Autodesk Fusion 360 part; units mm, degrees
note: some values were not read from the file. Chosen so that the rebuilt part matches the saved one: a direction. Set by a fixed rule: which sketch regions a step uses; which face or edge a step refers to.
(part 3 of 6)
  spline S532 degree 3 poles (194.827, -53.1151) (193.9004, -54.7201) (192.568, -56.0525) (190.963, -56.9791) knots 0 0 0 0 1 1 1 1
  spline S533 degree 3 poles (190.963, -56.9791) (189.3581, -57.9057) (187.5377, -58.3935) (185.6846, -58.3935) knots 0 0 0 0 1 1 1 1
  line L538 (185.6846, -58.3935) -> (156.5804, -58.3935)
  spline S534 degree 3 poles (156.5804, -58.3935) (156.5659, -58.3935) (156.554, -58.4054) (156.554, -58.42) knots 0 0 0 0 1 1 1 1
  line L539 (156.554, -58.42) -> (156.554, -59.2138)
  spline S535 degree 3 poles (156.554, -59.2138) (156.554, -59.2283) (156.5659, -59.2402) (156.5804, -59.2402) knots 0 0 0 0 1 1 1 1
  line L540 (155.3369, -57.9967) -> (184.441, -57.9967)
  spline S536 degree 3 poles (184.441, -57.9967) (186.4429, -57.9967) (188.4093, -57.4699) (190.1428, -56.469) knots 0 0 0 0 1 1 1 1
  spline S537 degree 3 poles (190.1428, -56.469) (191.8764, -55.468) (193.316, -54.0284) (194.3169, -52.2949) knots 0 0 0 0 1 1 1 1
  spline S538 degree 3 poles (194.3169, -52.2949) (195.3178, -50.5613) (195.8446, -48.595) (195.8446, -46.5931) knots 0 0 0 0 1 1 1 1
  spline S539 degree 3 poles (195.8446, -46.5931) (195.8446, -46.5786) (195.8327, -46.5667) (195.8181, -46.5667) knots 0 0 0 0 1 1 1 1
  line L541 (195.8181, -46.5667) -> (195.0244, -46.5667)
  spline S540 degree 3 poles (195.0244, -46.5667) (195.0098, -46.5667) (194.9979, -46.5786) (194.9979, -46.5931) knots 0 0 0 0 1 1 1 1
  spline S541 degree 3 poles (194.9979, -46.5931) (194.9979, -48.4463) (194.51, -50.2666) (193.5835, -51.8716) knots 0 0 0 0 1 1 1 1
  spline S542 degree 3 poles (193.5835, -51.8716) (192.6569, -53.4765) (191.3244, -54.809) (189.7195, -55.7355) knots 0 0 0 0 1 1 1 1
  spline S543 degree 3 poles (189.7195, -55.7355) (188.1145, -56.6621) (186.2942, -57.15) (184.441, -57.15) knots 0 0 0 0 1 1 1 1
  line L542 (184.441, -57.15) -> (155.3369, -57.15)
  spline S544 degree 3 poles (155.3369, -57.15) (155.3223, -57.15) (155.3104, -57.1619) (155.3104, -57.1765) knots 0 0 0 0 1 1 1 1
  line L543 (155.3104, -57.1765) -> (155.3104, -57.9702)
  spline S545 degree 3 poles (155.3104, -57.9702) (155.3104, -57.9848) (155.3223, -57.9967) (155.3369, -57.9967) knots 0 0 0 0 1 1 1 1
  line L544 (155.7337, -56.7531) -> (184.8379, -56.7531)
  spline S546 degree 3 poles (184.8379, -56.7531) (186.4913, -56.7531) (188.1156, -56.3179) (189.5475, -55.4913) knots 0 0 0 0 1 1 1 1
  spline S547 degree 3 poles (189.5475, -55.4913) (190.9794, -54.6645) (192.1685, -53.4755) (192.9953, -52.0435) knots 0 0 0 0 1 1 1 1
  spline S548 degree 3 poles (192.9953, -52.0435) (193.8218, -50.6116) (194.2571, -48.9873) (194.2571, -47.334) knots 0 0 0 0 1 1 1 1
  spline S549 degree 3 poles (194.2571, -47.334) (194.2571, -47.3194) (194.2452, -47.3075) (194.2306, -47.3075) knots 0 0 0 0 1 1 1 1
  line L545 (194.2306, -47.3075) -> (193.4369, -47.3075)
  spline S550 degree 3 poles (193.4369, -47.3075) (193.4223, -47.3075) (193.4104, -47.3194) (193.4104, -47.334) knots 0 0 0 0 1 1 1 1
  spline S551 degree 3 poles (193.4104, -47.334) (193.4104, -48.8386) (193.0143, -50.3171) (192.2619, -51.6202) knots 0 0 0 0 1 1 1 1
  spline S552 degree 3 poles (192.2619, -51.6202) (191.5096, -52.9233) (190.4272, -54.0057) (189.1242, -54.7579) knots 0 0 0 0 1 1 1 1
  spline S553 degree 3 poles (189.1242, -54.7579) (187.8211, -55.5104) (186.3426, -55.9065) (184.8379, -55.9065) knots 0 0 0 0 1 1 1 1
  line L546 (184.8379, -55.9065) -> (155.7337, -55.9065)
  spline S554 degree 3 poles (155.7337, -55.9065) (155.7192, -55.9065) (155.7073, -55.9184) (155.7073, -55.9329) knots 0 0 0 0 1 1 1 1
  line L547 (155.7073, -55.9329) -> (155.7073, -56.7267)
  spline S555 degree 3 poles (155.7073, -56.7267) (155.7073, -56.7412) (155.7192, -56.7531) (155.7337, -56.7531) knots 0 0 0 0 1 1 1 1
  line L548 (154.4902, -55.5096) -> (183.5944, -55.5096)
  spline S556 degree 3 poles (183.5944, -55.5096) (185.2478, -55.5096) (186.872, -55.0743) (188.304, -54.2478) knots 0 0 0 0 1 1 1 1
  spline S557 degree 3 poles (188.304, -54.2478) (189.7359, -53.421) (190.9249, -52.2319) (191.7517, -50.8) knots 0 0 0 0 1 1 1 1
  spline S558 degree 3 poles (191.7517, -50.8) (192.5783, -49.3681) (193.0135, -47.7438) (193.0135, -46.0904) knots 0 0 0 0 1 1 1 1
  spline S559 degree 3 poles (193.0135, -46.0904) (193.0135, -46.0759) (193.0016, -46.064) (192.9871, -46.064) knots 0 0 0 0 1 1 1 1
  line L549 (192.9871, -46.064) -> (192.1933, -46.064)
  spline S560 degree 3 poles (192.1933, -46.064) (192.1788, -46.064) (192.1669, -46.0759) (192.1669, -46.0904) knots 0 0 0 0 1 1 1 1
  spline S561 degree 3 poles (192.1669, -46.0904) (192.1669, -47.5951) (191.7708, -49.0736) (191.0183, -50.3767) knots 0 0 0 0 1 1 1 1
  spline S562 degree 3 poles (191.0183, -50.3767) (190.2661, -51.6797) (189.1837, -52.7622) (187.8806, -53.5144) knots 0 0 0 0 1 1 1 1
  spline S563 degree 3 poles (187.8806, -53.5144) (186.5775, -54.2668) (185.0991, -54.6629) (183.5944, -54.6629) knots 0 0 0 0 1 1 1 1
  line L550 (183.5944, -54.6629) -> (154.4902, -54.6629)
  spline S564 degree 3 poles (154.4902, -54.6629) (154.4756, -54.6629) (154.4637, -54.6748) (154.4637, -54.6894) knots 0 0 0 0 1 1 1 1
  line L551 (154.4637, -54.6894) -> (154.4637, -55.4831)
  spline S565 degree 3 poles (154.4637, -55.4831) (154.4637, -55.4977) (154.4756, -55.5096) (154.4902, -55.5096) knots 0 0 0 0 1 1 1 1
  line L552 (3.466, -30.7446) -> (5.0535, -30.7446)
  spline S566 degree 3 poles (5.0535, -30.7446) (5.0681, -30.7446) (5.08, -30.7327) (5.08, -30.7181) knots 0 0 0 0 1 1 1 1
  line L553 (5.08, -30.7181) -> (5.08, -29.9508)
  spline S567 degree 3 poles (5.08, -29.9508) (5.08, -29.9244) (5.0535, -29.9508) (5.08, -29.9508) knots 0 0 0 0 1 1 1 1
  line L554 (5.08, -29.9508) -> (6.6146, -29.9508)
  spline S568 degree 3 poles (6.6146, -29.9508) (6.641, -29.9508) (6.6146, -29.9244) (6.6146, -29.9508) knots 0 0 0 0 1 1 1 1
  line L555 (6.6146, -29.9508) -> (6.6146, -30.7181)
  spline S569 degree 3 poles (6.6146, -30.7181) (6.6146, -30.7327) (6.6265, -30.7446) (6.641, -30.7446) knots 0 0 0 0 1 1 1 1
  line L556 (6.641, -30.7446) -> (8.2285, -30.7446)
  spline S570 degree 3 poles (8.2285, -30.7446) (8.2431, -30.7446) (8.255, -30.7327) (8.255, -30.7181) knots 0 0 0 0 1 1 1 1
  line L557 (8.255, -30.7181) -> (8.255, -29.9508)
  spline S571 degree 3 poles (8.255, -29.9508) (8.255, -29.9244) (8.2285, -29.9508) (8.255, -29.9508) knots 0 0 0 0 1 1 1 1
  line L558 (8.255, -29.9508) -> (9.7896, -29.9508)
  spline S572 degree 3 poles (9.7896, -29.9508) (9.816, -29.9508) (9.7896, -29.9244) (9.7896, -29.9508) knots 0 0 0 0 1 1 1 1
  line L559 (9.7896, -29.9508) -> (9.7896, -30.7181)
  spline S573 degree 3 poles (9.7896, -30.7181) (9.7896, -30.7327) (9.8015, -30.7446) (9.816, -30.7446) knots 0 0 0 0 1 1 1 1
  line L560 (9.816, -30.7446) -> (11.4035, -30.7446)
  spline S574 degree 3 poles (11.4035, -30.7446) (11.4181, -30.7446) (11.43, -30.7327) (11.43, -30.7181) knots 0 0 0 0 1 1 1 1
  line L561 (11.43, -30.7181) -> (11.43, -29.9508)
  spline S575 degree 3 poles (11.43, -29.9508) (11.43, -29.9244) (11.4035, -29.9508) (11.43, -29.9508) knots 0 0 0 0 1 1 1 1
  line L562 (11.43, -29.9508) -> (12.9646, -29.9508)
  spline S576 degree 3 poles (12.9646, -29.9508) (12.991, -29.9508) (12.9646, -29.9244) (12.9646, -29.9508) knots 0 0 0 0 1 1 1 1
  line L563 (12.9646, -29.9508) -> (12.9646, -30.7181)
  spline S577 degree 3 poles (12.9646, -30.7181) (12.9646, -30.7327) (12.9765, -30.7446) (12.991, -30.7446) knots 0 0 0 0 1 1 1 1
  line L564 (12.991, -30.7446) -> (14.5785, -30.7446)
  spline S578 degree 3 poles (14.5785, -30.7446) (14.5931, -30.7446) (14.605, -30.7327) (14.605, -30.7181) knots 0 0 0 0 1 1 1 1
  line L565 (14.605, -30.7181) -> (14.605, -29.9508)
  spline S579 degree 3 poles (14.605, -29.9508) (14.605, -29.9244) (14.5785, -29.9508) (14.605, -29.9508) knots 0 0 0 0 1 1 1 1
  line L566 (14.605, -29.9508) -> (16.1396, -29.9508)
  spline S580 degree 3 poles (16.1396, -29.9508) (16.166, -29.9508) (16.1396, -29.9244) (16.1396, -29.9508) knots 0 0 0 0 1 1 1 1
  line L567 (16.1396, -29.9508) -> (16.1396, -30.7181)
  spline S581 degree 3 poles (16.1396, -30.7181) (16.1396, -30.7327) (16.1515, -30.7446) (16.166, -30.7446) knots 0 0 0 0 1 1 1 1
  line L568 (16.166, -30.7446) -> (17.7535, -30.7446)
  spline S582 degree 3 poles (17.7535, -30.7446) (17.7681, -30.7446) (17.78, -30.7327) (17.78, -30.7181) knots 0 0 0 0 1 1 1 1
  line L569 (17.78, -30.7181) -> (17.78, -29.9508)
  spline S583 degree 3 poles (17.78, -29.9508) (17.78, -29.9244) (17.7535, -29.9508) (17.78, -29.9508) knots 0 0 0 0 1 1 1 1
  line L570 (17.78, -29.9508) -> (19.3146, -29.9508)
  spline S584 degree 3 poles (19.3146, -29.9508) (19.341, -29.9508) (19.3146, -29.9244) (19.3146, -29.9508) knots 0 0 0 0 1 1 1 1
  line L571 (19.3146, -29.9508) -> (19.3146, -30.7181)
  spline S585 degree 3 poles (19.3146, -30.7181) (19.3146, -30.7327) (19.3265, -30.7446) (19.341, -30.7446) knots 0 0 0 0 1 1 1 1
  line L572 (19.341, -30.7446) -> (20.9285, -30.7446)
  spline S586 degree 3 poles (20.9285, -30.7446) (20.9431, -30.7446) (20.955, -30.7327) (20.955, -30.7181) knots 0 0 0 0 1 1 1 1
  line L573 (20.955, -30.7181) -> (20.955, -29.9508)
  spline S587 degree 3 poles (20.955, -29.9508) (20.955, -29.9244) (20.9285, -29.9508) (20.955, -29.9508) knots 0 0 0 0 1 1 1 1
  line L574 (20.955, -29.9508) -> (22.4896, -29.9508)
  spline S588 degree 3 poles (22.4896, -29.9508) (22.516, -29.9508) (22.4896, -29.9244) (22.4896, -29.9508) knots 0 0 0 0 1 1 1 1
  line L575 (22.4896, -29.9508) -> (22.4896, -30.7181)
  spline S589 degree 3 poles (22.4896, -30.7181) (22.4896, -30.7327) (22.5015, -30.7446) (22.516, -30.7446) knots 0 0 0 0 1 1 1 1
  line L576 (22.516, -30.7446) -> (24.1035, -30.7446)
  spline S590 degree 3 poles (24.1035, -30.7446) (24.1181, -30.7446) (24.13, -30.7327) (24.13, -30.7181) knots 0 0 0 0 1 1 1 1
  line L577 (24.13, -30.7181) -> (24.13, -29.9508)
  spline S591 degree 3 poles (24.13, -29.9508) (24.13, -29.9244) (24.1035, -29.9508) (24.13, -29.9508) knots 0 0 0 0 1 1 1 1
  line L578 (24.13, -29.9508) -> (25.6646, -29.9508)
  spline S592 degree 3 poles (25.6646, -29.9508) (25.691, -29.9508) (25.6646, -29.9244) (25.6646, -29.9508) knots 0 0 0 0 1 1 1 1
  line L579 (25.6646, -29.9508) -> (25.6646, -30.7181)
  spline S593 degree 3 poles (25.6646, -30.7181) (25.6646, -30.7327) (25.6765, -30.7446) (25.691, -30.7446) knots 0 0 0 0 1 1 1 1
  line L580 (25.691, -30.7446) -> (27.2785, -30.7446)
  spline S594 degree 3 poles (27.2785, -30.7446) (27.2931, -30.7446) (27.305, -30.7327) (27.305, -30.7181) knots 0 0 0 0 1 1 1 1
  line L581 (27.305, -30.7181) -> (27.305, -29.9508)
  spline S595 degree 3 poles (27.305, -29.9508) (27.305, -29.9244) (27.2785, -29.9508) (27.305, -29.9508) knots 0 0 0 0 1 1 1 1
  line L582 (27.305, -29.9508) -> (28.8396, -29.9508)
  spline S596 degree 3 poles (28.8396, -29.9508) (28.866, -29.9508) (28.8396, -29.9244) (28.8396, -29.9508) knots 0 0 0 0 1 1 1 1
  line L583 (28.8396, -29.9508) -> (28.8396, -30.7181)
  spline S597 degree 3 poles (28.8396, -30.7181) (28.8396, -30.7327) (28.8515, -30.7446) (28.866, -30.7446) knots 0 0 0 0 1 1 1 1
  line L584 (28.866, -30.7446) -> (30.4535, -30.7446)
  spline S598 degree 3 poles (30.4535, -30.7446) (30.4681, -30.7446) (30.48, -30.7327) (30.48, -30.7181) knots 0 0 0 0 1 1 1 1
  line L585 (30.48, -30.7181) -> (30.48, -29.9508)
  spline S599 degree 3 poles (30.48, -29.9508) (30.48, -29.9244) (30.4535, -29.9508) (30.48, -29.9508) knots 0 0 0 0 1 1 1 1
  line L586 (30.48, -29.9508) -> (32.0146, -29.9508)
  spline S600 degree 3 poles (32.0146, -29.9508) (32.041, -29.9508) (32.0146, -29.9244) (32.0146, -29.9508) knots 0 0 0 0 1 1 1 1
  line L587 (32.0146, -29.9508) -> (32.0146, -30.7181)
  spline S601 degree 3 poles (32.0146, -30.7181) (32.0146, -30.7327) (32.0265, -30.7446) (32.041, -30.7446) knots 0 0 0 0 1 1 1 1
  line L588 (32.041, -30.7446) -> (33.6285, -30.7446)
  spline S602 degree 3 poles (33.6285, -30.7446) (33.6431, -30.7446) (33.655, -30.7327) (33.655, -30.7181) knots 0 0 0 0 1 1 1 1
  line L589 (33.655, -30.7181) -> (33.655, -29.9508)
  spline S603 degree 3 poles (33.655, -29.9508) (33.655, -29.9244) (33.6285, -29.9508) (33.655, -29.9508) knots 0 0 0 0 1 1 1 1
  line L590 (33.655, -29.9508) -> (35.1896, -29.9508)
  spline S604 degree 3 poles (35.1896, -29.9508) (35.216, -29.9508) (35.1896, -29.9244) (35.1896, -29.9508) knots 0 0 0 0 1 1 1 1
  line L591 (35.1896, -29.9508) -> (35.1896, -30.7181)
  spline S605 degree 3 poles (35.1896, -30.7181) (35.1896, -30.7327) (35.2015, -30.7446) (35.216, -30.7446) knots 0 0 0 0 1 1 1 1
  line L592 (35.216, -30.7446) -> (36.8035, -30.7446)
  spline S606 degree 3 poles (36.8035, -30.7446) (36.8181, -30.7446) (36.83, -30.7327) (36.83, -30.7181) knots 0 0 0 0 1 1 1 1
  line L593 (36.83, -30.7181) -> (36.83, -29.9508)
  spline S607 degree 3 poles (36.83, -29.9508) (36.83, -29.9244) (36.8035, -29.9508) (36.83, -29.9508) knots 0 0 0 0 1 1 1 1
  line L594 (36.83, -29.9508) -> (38.3646, -29.9508)
  spline S608 degree 3 poles (38.3646, -29.9508) (38.391, -29.9508) (38.3646, -29.9244) (38.3646, -29.9508) knots 0 0 0 0 1 1 1 1
  line L595 (38.3646, -29.9508) -> (38.3646, -30.7181)
  spline S609 degree 3 poles (38.3646, -30.7181) (38.3646, -30.7327) (38.3765, -30.7446) (38.391, -30.7446) knots 0 0 0 0 1 1 1 1
  line L596 (38.391, -30.7446) -> (39.9785, -30.7446)
  spline S610 degree 3 poles (39.9785, -30.7446) (39.9931, -30.7446) (40.005, -30.7327) (40.005, -30.7181) knots 0 0 0 0 1 1 1 1
  line L597 (40.005, -30.7181) -> (40.005, -29.9508)
  spline S611 degree 3 poles (40.005, -29.9508) (40.005, -29.9244) (39.9785, -29.9508) (40.005, -29.9508) knots 0 0 0 0 1 1 1 1
  line L598 (40.005, -29.9508) -> (41.5396, -29.9508)
  spline S612 degree 3 poles (41.5396, -29.9508) (41.566, -29.9508) (41.5396, -29.9244) (41.5396, -29.9508) knots 0 0 0 0 1 1 1 1
  line L599 (41.5396, -29.9508) -> (41.5396, -30.7181)
  spline S613 degree 3 poles (41.5396, -30.7181) (41.5396, -30.7327) (41.5515, -30.7446) (41.566, -30.7446) knots 0 0 0 0 1 1 1 1
  line L600 (41.566, -30.7446) -> (43.1535, -30.7446)
  line L601 (43.1535, -30.7446) -> (43.9473, -30.7446)
  spline S614 degree 3 poles (43.9473, -30.7446) (43.9618, -30.7446) (43.9737, -30.7327) (43.9737, -30.7181) knots 0 0 0 0 1 1 1 1
  line L602 (43.9737, -30.7181) -> (43.9737, -29.9244)
  line L603 (43.9737, -29.9244) -> (43.9737, -28.6015)
  spline S615 degree 3 poles (43.9737, -28.6015) (43.9737, -28.5869) (43.9618, -28.575) (43.9473, -28.575) knots 0 0 0 0 1 1 1 1
  line L604 (43.9473, -28.575) -> (43.18, -28.575)
  spline S616 degree 3 poles (43.18, -28.575) (43.1535, -28.575) (43.18, -28.6015) (43.18, -28.575) knots 0 0 0 0 1 1 1 1
  line L605 (43.18, -28.575) -> (43.18, -27.0404)
  spline S617 degree 3 poles (43.18, -27.0404) (43.18, -27.014) (43.1535, -27.0404) (43.18, -27.0404) knots 0 0 0 0 1 1 1 1
  line L606 (43.18, -27.0404) -> (43.9473, -27.0404)
  spline S618 degree 3 poles (43.9473, -27.0404) (43.9618, -27.0404) (43.9737, -27.0285) (43.9737, -27.014) knots 0 0 0 0 1 1 1 1
  line L607 (43.9737, -27.014) -> (43.9737, -25.4265)
  spline S619 degree 3 poles (43.9737, -25.4265) (43.9737, -25.4119) (43.9618, -25.4) (43.9473, -25.4) knots 0 0 0 0 1 1 1 1
  line L608 (43.9473, -25.4) -> (43.18, -25.4)
  spline S620 degree 3 poles (43.18, -25.4) (43.1535, -25.4) (43.18, -25.4265) (43.18, -25.4) knots 0 0 0 0 1 1 1 1
  line L609 (43.18, -25.4) -> (43.18, -23.8654)
  spline S621 degree 3 poles (43.18, -23.8654) (43.18, -23.839) (43.1535, -23.8654) (43.18, -23.8654) knots 0 0 0 0 1 1 1 1
  line L610 (43.18, -23.8654) -> (43.9473, -23.8654)
  spline S622 degree 3 poles (43.9473, -23.8654) (43.9618, -23.8654) (43.9737, -23.8535) (43.9737, -23.839) knots 0 0 0 0 1 1 1 1
  line L611 (43.9737, -23.839) -> (43.9737, -22.2515)
  spline S623 degree 3 poles (43.9737, -22.2515) (43.9737, -22.2369) (43.9618, -22.225) (43.9473, -22.225) knots 0 0 0 0 1 1 1 1
  line L612 (43.9473, -22.225) -> (43.18, -22.225)
  spline S624 degree 3 poles (43.18, -22.225) (43.1535, -22.225) (43.18, -22.2515) (43.18, -22.225) knots 0 0 0 0 1 1 1 1
  line L613 (43.18, -22.225) -> (43.18, -20.6904)
  spline S625 degree 3 poles (43.18, -20.6904) (43.18, -20.664) (43.1535, -20.6904) (43.18, -20.6904) knots 0 0 0 0 1 1 1 1
  line L614 (43.18, -20.6904) -> (43.9473, -20.6904)
  spline S626 degree 3 poles (43.9473, -20.6904) (43.9618, -20.6904) (43.9737, -20.6785) (43.9737, -20.664) knots 0 0 0 0 1 1 1 1
  line L615 (43.9737, -20.664) -> (43.9737, -19.0765)
  spline S627 degree 3 poles (43.9737, -19.0765) (43.9737, -19.0619) (43.9618, -19.05) (43.9473, -19.05) knots 0 0 0 0 1 1 1 1
  line L616 (43.9473, -19.05) -> (43.18, -19.05)
  spline S628 degree 3 poles (43.18, -19.05) (43.1535, -19.05) (43.18, -19.0765) (43.18, -19.05) knots 0 0 0 0 1 1 1 1
  line L617 (43.18, -19.05) -> (43.18, -17.5154)
  spline S629 degree 3 poles (43.18, -17.5154) (43.18, -17.489) (43.1535, -17.5154) (43.18, -17.5154) knots 0 0 0 0 1 1 1 1
  line L618 (43.18, -17.5154) -> (43.9473, -17.5154)
  spline S630 degree 3 poles (43.9473, -17.5154) (43.9618, -17.5154) (43.9737, -17.5035) (43.9737, -17.489) knots 0 0 0 0 1 1 1 1
  line L619 (43.9737, -17.489) -> (43.9737, -15.9015)
  spline S631 degree 3 poles (43.9737, -15.9015) (43.9737, -15.8869) (43.9618, -15.875) (43.9473, -15.875) knots 0 0 0 0 1 1 1 1
  line L620 (43.9473, -15.875) -> (43.18, -15.875)
  spline S632 degree 3 poles (43.18, -15.875) (43.1535, -15.875) (43.18, -15.9015) (43.18, -15.875) knots 0 0 0 0 1 1 1 1
  line L621 (43.18, -15.875) -> (43.18, -14.3404)
  spline S633 degree 3 poles (43.18, -14.3404) (43.18, -14.314) (43.1535, -14.3404) (43.18, -14.3404) knots 0 0 0 0 1 1 1 1
  line L622 (43.18, -14.3404) -> (43.9473, -14.3404)
  spline S634 degree 3 poles (43.9473, -14.3404) (43.9618, -14.3404) (43.9737, -14.3285) (43.9737, -14.314) knots 0 0 0 0 1 1 1 1
  line L623 (43.9737, -14.314) -> (43.9737, -12.7265)
  spline S635 degree 3 poles (43.9737, -12.7265) (43.9737, -12.7119) (43.9618, -12.7) (43.9473, -12.7) knots 0 0 0 0 1 1 1 1
  line L624 (43.9473, -12.7) -> (43.18, -12.7)
  spline S636 degree 3 poles (43.18, -12.7) (43.1535, -12.7) (43.18, -12.7265) (43.18, -12.7) knots 0 0 0 0 1 1 1 1
  line L625 (43.18, -12.7) -> (43.18, -11.1654)
  spline S637 degree 3 poles (43.18, -11.1654) (43.18, -11.139) (43.1535, -11.1654) (43.18, -11.1654) knots 0 0 0 0 1 1 1 1
  line L626 (43.18, -11.1654) -> (43.9473, -11.1654)
  spline S638 degree 3 poles (43.9473, -11.1654) (43.9618, -11.1654) (43.9737, -11.1535) (43.9737, -11.139) knots 0 0 0 0 1 1 1 1
  line L627 (43.9737, -11.139) -> (43.9737, -9.5515)
  spline S639 degree 3 poles (43.9737, -9.5515) (43.9737, -9.5369) (43.9618, -9.525) (43.9473, -9.525) knots 0 0 0 0 1 1 1 1
  line L628 (43.9473, -9.525) -> (43.18, -9.525)
  spline S640 degree 3 poles (43.18, -9.525) (43.1535, -9.525) (43.18, -9.5515) (43.18, -9.525) knots 0 0 0 0 1 1 1 1
  line L629 (43.18, -9.525) -> (43.18, -7.9904)
  spline S641 degree 3 poles (43.18, -7.9904) (43.18, -7.964) (43.1535, -7.9904) (43.18, -7.9904) knots 0 0 0 0 1 1 1 1
  line L630 (43.18, -7.9904) -> (43.9473, -7.9904)
  spline S642 degree 3 poles (43.9473, -7.9904) (43.9618, -7.9904) (43.9737, -7.9785) (43.9737, -7.964) knots 0 0 0 0 1 1 1 1
  line L631 (43.9737, -7.964) -> (43.9737, -6.3765)
  spline S643 degree 3 poles (43.9737, -6.3765) (43.9737, -6.3619) (43.9618, -6.35) (43.9473, -6.35) knots 0 0 0 0 1 1 1 1
  line L632 (43.9473, -6.35) -> (43.18, -6.35)
  spline S644 degree 3 poles (43.18, -6.35) (43.1535, -6.35) (43.18, -6.3765) (43.18, -6.35) knots 0 0 0 0 1 1 1 1
  line L633 (43.18, -6.35) -> (43.18, -4.8154)
  spline S645 degree 3 poles (43.18, -4.8154) (43.18, -4.789) (43.1535, -4.8154) (43.18, -4.8154) knots 0 0 0 0 1 1 1 1
  line L634 (43.18, -4.8154) -> (43.9473, -4.8154)
  spline S646 degree 3 poles (43.9473, -4.8154) (43.9618, -4.8154) (43.9737, -4.8035) (43.9737, -4.789) knots 0 0 0 0 1 1 1 1
  line L635 (43.9737, -4.789) -> (43.9737, -3.466)
  line L636 (43.9737, -3.466) -> (43.9737, -2.6723)
  spline S647 degree 3 poles (43.9737, -2.6723) (43.9737, -2.6577) (43.9618, -2.6458) (43.9473, -2.6458) knots 0 0 0 0 1 1 1 1
  line L637 (43.9473, -2.6458) -> (43.1535, -2.6458)
  line L638 (43.1535, -2.6458) -> (41.566, -2.6458)
  spline S648 degree 3 poles (41.566, -2.6458) (41.5515, -2.6458) (41.5396, -2.6577) (41.5396, -2.6723) knots 0 0 0 0 1 1 1 1
  line L639 (41.5396, -2.6723) -> (41.5396, -3.4396)
  spline S649 degree 3 poles (41.5396, -3.4396) (41.5396, -3.466) (41.566, -3.4396) (41.5396, -3.4396) knots 0 0 0 0 1 1 1 1
  line L640 (41.5396, -3.4396) -> (40.005, -3.4396)
  spline S650 degree 3 poles (40.005, -3.4396) (39.9785, -3.4396) (40.005, -3.466) (40.005, -3.4396) knots 0 0 0 0 1 1 1 1
  line L641 (40.005, -3.4396) -> (40.005, -2.6723)
  spline S651 degree 3 poles (40.005, -2.6723) (40.005, -2.6577) (39.9931, -2.6458) (39.9785, -2.6458) knots 0 0 0 0 1 1 1 1
  line L642 (39.9785, -2.6458) -> (38.391, -2.6458)
  spline S652 degree 3 poles (38.391, -2.6458) (38.3765, -2.6458) (38.3646, -2.6577) (38.3646, -2.6723) knots 0 0 0 0 1 1 1 1
  line L643 (38.3646, -2.6723) -> (38.3646, -3.4396)
  spline S653 degree 3 poles (38.3646, -3.4396) (38.3646, -3.466) (38.391, -3.4396) (38.3646, -3.4396) knots 0 0 0 0 1 1 1 1
  line L644 (38.3646, -3.4396) -> (36.83, -3.4396)
  spline S654 degree 3 poles (36.83, -3.4396) (36.8035, -3.4396) (36.83, -3.466) (36.83, -3.4396) knots 0 0 0 0 1 1 1 1
  line L645 (36.83, -3.4396) -> (36.83, -2.6723)
  spline S655 degree 3 poles (36.83, -2.6723) (36.83, -2.6577) (36.8181, -2.6458) (36.8035, -2.6458) knots 0 0 0 0 1 1 1 1
  line L646 (36.8035, -2.6458) -> (35.216, -2.6458)
  spline S656 degree 3 poles (35.216, -2.6458) (35.2015, -2.6458) (35.1896, -2.6577) (35.1896, -2.6723) knots 0 0 0 0 1 1 1 1
  line L647 (35.1896, -2.6723) -> (35.1896, -3.4396)
  spline S657 degree 3 poles (35.1896, -3.4396) (35.1896, -3.466) (35.216, -3.4396) (35.1896, -3.4396) knots 0 0 0 0 1 1 1 1
  line L648 (35.1896, -3.4396) -> (33.655, -3.4396)
  spline S658 degree 3 poles (33.655, -3.4396) (33.6285, -3.4396) (33.655, -3.466) (33.655, -3.4396) knots 0 0 0 0 1 1 1 1
  line L649 (33.655, -3.4396) -> (33.655, -2.6723)
  spline S659 degree 3 poles (33.655, -2.6723) (33.655, -2.6577) (33.6431, -2.6458) (33.6285, -2.6458) knots 0 0 0 0 1 1 1 1
  line L650 (33.6285, -2.6458) -> (32.041, -2.6458)
  spline S660 degree 3 poles (32.041, -2.6458) (32.0265, -2.6458) (32.0146, -2.6577) (32.0146, -2.6723) knots 0 0 0 0 1 1 1 1
  line L651 (32.0146, -2.6723) -> (32.0146, -3.4396)
  spline S661 degree 3 poles (32.0146, -3.4396) (32.0146, -3.466) (32.041, -3.4396) (32.0146, -3.4396) knots 0 0 0 0 1 1 1 1
  line L652 (32.0146, -3.4396) -> (30.48, -3.4396)
  spline S662 degree 3 poles (30.48, -3.4396) (30.4535, -3.4396) (30.48, -3.466) (30.48, -3.4396) knots 0 0 0 0 1 1 1 1
  line L653 (30.48, -3.4396) -> (30.48, -2.6723)
  spline S663 degree 3 poles (30.48, -2.6723) (30.48, -2.6577) (30.4681, -2.6458) (30.4535, -2.6458) knots 0 0 0 0 1 1 1 1
  line L654 (30.4535, -2.6458) -> (28.866, -2.6458)
  spline S664 degree 3 poles (28.866, -2.6458) (28.8515, -2.6458) (28.8396, -2.6577) (28.8396, -2.6723) knots 0 0 0 0 1 1 1 1
  line L655 (28.8396, -2.6723) -> (28.8396, -3.4396)
  spline S665 degree 3 poles (28.8396, -3.4396) (28.8396, -3.466) (28.866, -3.4396) (28.8396, -3.4396) knots 0 0 0 0 1 1 1 1
  line L656 (28.8396, -3.4396) -> (27.305, -3.4396)
  spline S666 degree 3 poles (27.305, -3.4396) (27.2785, -3.4396) (27.305, -3.466) (27.305, -3.4396) knots 0 0 0 0 1 1 1 1
  line L657 (27.305, -3.4396) -> (27.305, -2.6723)
  spline S667 degree 3 poles (27.305, -2.6723) (27.305, -2.6577) (27.2931, -2.6458) (27.2785, -2.6458) knots 0 0 0 0 1 1 1 1
  line L658 (27.2785, -2.6458) -> (25.691, -2.6458)
  spline S668 degree 3 poles (25.691, -2.6458) (25.6765, -2.6458) (25.6646, -2.6577) (25.6646, -2.6723) knots 0 0 0 0 1 1 1 1
  line L659 (25.6646, -2.6723) -> (25.6646, -3.4396)
  spline S669 degree 3 poles (25.6646, -3.4396) (25.6646, -3.466) (25.691, -3.4396) (25.6646, -3.4396) knots 0 0 0 0 1 1 1 1
  line L660 (25.6646, -3.4396) -> (24.13, -3.4396)
  spline S670 degree 3 poles (24.13, -3.4396) (24.1035, -3.4396) (24.13, -3.466) (24.13, -3.4396) knots 0 0 0 0 1 1 1 1
  line L661 (24.13, -3.4396) -> (24.13, -2.6723)
  spline S671 degree 3 poles (24.13, -2.6723) (24.13, -2.6577) (24.1181, -2.6458) (24.1035, -2.6458) knots 0 0 0 0 1 1 1 1
  line L662 (24.1035, -2.6458) -> (22.516, -2.6458)
  spline S672 degree 3 poles (22.516, -2.6458) (22.5015, -2.6458) (22.4896, -2.6577) (22.4896, -2.6723) knots 0 0 0 0 1 1 1 1
  line L663 (22.4896, -2.6723) -> (22.4896, -3.4396)
  spline S673 degree 3 poles (22.4896, -3.4396) (22.4896, -3.466) (22.516, -3.4396) (22.4896, -3.4396) knots 0 0 0 0 1 1 1 1
  line L664 (22.4896, -3.4396) -> (20.955, -3.4396)
  spline S674 degree 3 poles (20.955, -3.4396) (20.9285, -3.4396) (20.955, -3.466) (20.955, -3.4396) knots 0 0 0 0 1 1 1 1
  line L665 (20.955, -3.4396) -> (20.955, -2.6723)
  spline S675 degree 3 poles (20.955, -2.6723) (20.955, -2.6577) (20.9431, -2.6458) (20.9285, -2.6458) knots 0 0 0 0 1 1 1 1
  line L666 (20.9285, -2.6458) -> (19.341, -2.6458)
  spline S676 degree 3 poles (19.341, -2.6458) (19.3265, -2.6458) (19.3146, -2.6577) (19.3146, -2.6723) knots 0 0 0 0 1 1 1 1
  line L667 (19.3146, -2.6723) -> (19.3146, -3.4396)
  spline S677 degree 3 poles (19.3146, -3.4396) (19.3146, -3.466) (19.341, -3.4396) (19.3146, -3.4396) knots 0 0 0 0 1 1 1 1
  line L668 (19.3146, -3.4396) -> (17.78, -3.4396)
  spline S678 degree 3 poles (17.78, -3.4396) (17.7535, -3.4396) (17.78, -3.466) (17.78, -3.4396) knots 0 0 0 0 1 1 1 1
  line L669 (17.78, -3.4396) -> (17.78, -2.6723)
  spline S679 degree 3 poles (17.78, -2.6723) (17.78, -2.6577) (17.7681, -2.6458) (17.7535, -2.6458) knots 0 0 0 0 1 1 1 1
  line L670 (17.7535, -2.6458) -> (16.166, -2.6458)
  spline S680 degree 3 poles (16.166, -2.6458) (16.1515, -2.6458) (16.1396, -2.6577) (16.1396, -2.6723) knots 0 0 0 0 1 1 1 1
  line L671 (16.1396, -2.6723) -> (16.1396, -3.4396)
  spline S681 degree 3 poles (16.1396, -3.4396) (16.1396, -3.466) (16.166, -3.4396) (16.1396, -3.4396) knots 0 0 0 0 1 1 1 1
  line L672 (16.1396, -3.4396) -> (14.605, -3.4396)
  spline S682 degree 3 poles (14.605, -3.4396) (14.5785, -3.4396) (14.605, -3.466) (14.605, -3.4396) knots 0 0 0 0 1 1 1 1
  line L673 (14.605, -3.4396) -> (14.605, -2.6723)
  spline S683 degree 3 poles (14.605, -2.6723) (14.605, -2.6577) (14.5931, -2.6458) (14.5785, -2.6458) knots 0 0 0 0 1 1 1 1
  line L674 (14.5785, -2.6458) -> (12.991, -2.6458)
  spline S684 degree 3 poles (12.991, -2.6458) (12.9765, -2.6458) (12.9646, -2.6577) (12.9646, -2.6723) knots 0 0 0 0 1 1 1 1
  line L675 (12.9646, -2.6723) -> (12.9646, -3.4396)
  spline S685 degree 3 poles (12.9646, -3.4396) (12.9646, -3.466) (12.991, -3.4396) (12.9646, -3.4396) knots 0 0 0 0 1 1 1 1
  line L676 (12.9646, -3.4396) -> (11.43, -3.4396)
  spline S686 degree 3 poles (11.43, -3.4396) (11.4035, -3.4396) (11.43, -3.466) (11.43, -3.4396) knots 0 0 0 0 1 1 1 1
  line L677 (11.43, -3.4396) -> (11.43, -2.6723)
  spline S687 degree 3 poles (11.43, -2.6723) (11.43, -2.6577) (11.4181, -2.6458) (11.4035, -2.6458) knots 0 0 0 0 1 1 1 1
  line L678 (11.4035, -2.6458) -> (9.816, -2.6458)
  spline S688 degree 3 poles (9.816, -2.6458) (9.8015, -2.6458) (9.7896, -2.6577) (9.7896, -2.6723) knots 0 0 0 0 1 1 1 1
  line L679 (9.7896, -2.6723) -> (9.7896, -3.4396)
  spline S689 degree 3 poles (9.7896, -3.4396) (9.7896, -3.466) (9.816, -3.4396) (9.7896, -3.4396) knots 0 0 0 0 1 1 1 1
  line L680 (9.7896, -3.4396) -> (8.255, -3.4396)
  spline S690 degree 3 poles (8.255, -3.4396) (8.2285, -3.4396) (8.255, -3.466) (8.255, -3.4396) knots 0 0 0 0 1 1 1 1
  line L681 (8.255, -3.4396) -> (8.255, -2.6723)
  spline S691 degree 3 poles (8.255, -2.6723) (8.255, -2.6577) (8.2431, -2.6458) (8.2285, -2.6458) knots 0 0 0 0 1 1 1 1
  line L682 (8.2285, -2.6458) -> (6.641, -2.6458)
  spline S692 degree 3 poles (6.641, -2.6458) (6.6265, -2.6458) (6.6146, -2.6577) (6.6146, -2.6723) knots 0 0 0 0 1 1 1 1
  line L683 (6.6146, -2.6723) -> (6.6146, -3.4396)
  spline S693 degree 3 poles (6.6146, -3.4396) (6.6146, -3.466) (6.641, -3.4396) (6.6146, -3.4396) knots 0 0 0 0 1 1 1 1
  line L684 (6.6146, -3.4396) -> (5.08, -3.4396)
  spline S694 degree 3 poles (5.08, -3.4396) (5.0535, -3.4396) (5.08, -3.466) (5.08, -3.4396) knots 0 0 0 0 1 1 1 1
  line L685 (5.08, -3.4396) -> (5.08, -2.6723)
  spline S695 degree 3 poles (5.08, -2.6723) (5.08, -2.6577) (5.0681, -2.6458) (5.0535, -2.6458) knots 0 0 0 0 1 1 1 1
  line L686 (5.0535, -2.6458) -> (3.466, -2.6458)
  line L687 (3.466, -2.6458) -> (2.6723, -2.6458)
  spline S696 degree 3 poles (2.6723, -2.6458) (2.6577, -2.6458) (2.6458, -2.6577) (2.6458, -2.6723) knots 0 0 0 0 1 1 1 1
  line L688 (2.6458, -2.6723) -> (2.6458, -3.466)
  line L689 (2.6458, -3.466) -> (2.6458, -4.789)
  spline S697 degree 3 poles (2.6458, -4.789) (2.6458, -4.8035) (2.6577, -4.8154) (2.6723, -4.8154) knots 0 0 0 0 1 1 1 1
  line L690 (2.6723, -4.8154) -> (3.4396, -4.8154)
  spline S698 degree 3 poles (3.4396, -4.8154) (3.466, -4.8154) (3.4396, -4.789) (3.4396, -4.8154) knots 0 0 0 0 1 1 1 1
  line L691 (3.4396, -4.8154) -> (3.4396, -6.35)
  spline S699 degree 3 poles (3.4396, -6.35) (3.4396, -6.3765) (3.466, -6.35) (3.4396, -6.35) knots 0 0 0 0 1 1 1 1
  line L692 (3.4396, -6.35) -> (2.6723, -6.35)
  spline S700 degree 3 poles (2.6723, -6.35) (2.6577, -6.35) (2.6458, -6.3619) (2.6458, -6.3765) knots 0 0 0 0 1 1 1 1
  line L693 (2.6458, -6.3765) -> (2.6458, -7.964)
  spline S701 degree 3 poles (2.6458, -7.964) (2.6458, -7.9785) (2.6577, -7.9904) (2.6723, -7.9904) knots 0 0 0 0 1 1 1 1
  line L694 (2.6723, -7.9904) -> (3.4396, -7.9904)
  spline S702 degree 3 poles (3.4396, -7.9904) (3.466, -7.9904) (3.4396, -7.964) (3.4396, -7.9904) knots 0 0 0 0 1 1 1 1
  line L695 (3.4396, -7.9904) -> (3.4396, -9.525)
  spline S703 degree 3 poles (3.4396, -9.525) (3.4396, -9.5515) (3.466, -9.525) (3.4396, -9.525) knots 0 0 0 0 1 1 1 1
  line L696 (3.4396, -9.525) -> (2.6723, -9.525)
  spline S704 degree 3 poles (2.6723, -9.525) (2.6577, -9.525) (2.6458, -9.5369) (2.6458, -9.5515) knots 0 0 0 0 1 1 1 1
  line L697 (2.6458, -9.5515) -> (2.6458, -11.139)
  spline S705 degree 3 poles (2.6458, -11.139) (2.6458, -11.1535) (2.6577, -11.1654) (2.6723, -11.1654) knots 0 0 0 0 1 1 1 1
  line L698 (2.6723, -11.1654) -> (3.4396, -11.1654)
  spline S706 degree 3 poles (3.4396, -11.1654) (3.466, -11.1654) (3.4396, -11.139) (3.4396, -11.1654) knots 0 0 0 0 1 1 1 1
  line L699 (3.4396, -11.1654) -> (3.4396, -12.7)
  spline S707 degree 3 poles (3.4396, -12.7) (3.4396, -12.7265) (3.466, -12.7) (3.4396, -12.7) knots 0 0 0 0 1 1 1 1
  line L700 (3.4396, -12.7) -> (2.6723, -12.7)
  spline S708 degree 3 poles (2.6723, -12.7) (2.6577, -12.7) (2.6458, -12.7119) (2.6458, -12.7265) knots 0 0 0 0 1 1 1 1
  line L701 (2.6458, -12.7265) -> (2.6458, -14.314)
  spline S709 degree 3 poles (2.6458, -14.314) (2.6458, -14.3285) (2.6577, -14.3404) (2.6723, -14.3404) knots 0 0 0 0 1 1 1 1
  line L702 (2.6723, -14.3404) -> (3.4396, -14.3404)
  spline S710 degree 3 poles (3.4396, -14.3404) (3.466, -14.3404) (3.4396, -14.314) (3.4396, -14.3404) knots 0 0 0 0 1 1 1 1
  line L703 (3.4396, -14.3404) -> (3.4396, -15.875)
  spline S711 degree 3 poles (3.4396, -15.875) (3.4396, -15.9015) (3.466, -15.875) (3.4396, -15.875) knots 0 0 0 0 1 1 1 1
  line L704 (3.4396, -15.875) -> (2.6723, -15.875)
  spline S712 degree 3 poles (2.6723, -15.875) (2.6577, -15.875) (2.6458, -15.8869) (2.6458, -15.9015) knots 0 0 0 0 1 1 1 1
  line L705 (2.6458, -15.9015) -> (2.6458, -17.489)
  spline S713 degree 3 poles (2.6458, -17.489) (2.6458, -17.5035) (2.6577, -17.5154) (2.6723, -17.5154) knots 0 0 0 0 1 1 1 1
  line L706 (2.6723, -17.5154) -> (3.4396, -17.5154)
  spline S714 degree 3 poles (3.4396, -17.5154) (3.466, -17.5154) (3.4396, -17.489) (3.4396, -17.5154) knots 0 0 0 0 1 1 1 1
  line L707 (3.4396, -17.5154) -> (3.4396, -19.05)
  spline S715 degree 3 poles (3.4396, -19.05) (3.4396, -19.0765) (3.466, -19.05) (3.4396, -19.05) knots 0 0 0 0 1 1 1 1
  line L708 (3.4396, -19.05) -> (2.6723, -19.05)
  spline S716 degree 3 poles (2.6723, -19.05) (2.6577, -19.05) (2.6458, -19.0619) (2.6458, -19.0765) knots 0 0 0 0 1 1 1 1
  line L709 (2.6458, -19.0765) -> (2.6458, -20.664)
  spline S717 degree 3 poles (2.6458, -20.664) (2.6458, -20.6785) (2.6577, -20.6904) (2.6723, -20.6904) knots 0 0 0 0 1 1 1 1
  line L710 (2.6723, -20.6904) -> (3.4396, -20.6904)
  spline S718 degree 3 poles (3.4396, -20.6904) (3.466, -20.6904) (3.4396, -20.664) (3.4396, -20.6904) knots 0 0 0 0 1 1 1 1
  line L711 (3.4396, -20.6904) -> (3.4396, -22.225)
  spline S719 degree 3 poles (3.4396, -22.225) (3.4396, -22.2515) (3.466, -22.225) (3.4396, -22.225) knots 0 0 0 0 1 1 1 1
  line L712 (3.4396, -22.225) -> (2.6723, -22.225)
  spline S720 degree 3 poles (2.6723, -22.225) (2.6577, -22.225) (2.6458, -22.2369) (2.6458, -22.2515) knots 0 0 0 0 1 1 1 1
  line L713 (2.6458, -22.2515) -> (2.6458, -23.839)
  spline S721 degree 3 poles (2.6458, -23.839) (2.6458, -23.8535) (2.6577, -23.8654) (2.6723, -23.8654) knots 0 0 0 0 1 1 1 1
  line L714 (2.6723, -23.8654) -> (3.4396, -23.8654)
  spline S722 degree 3 poles (3.4396, -23.8654) (3.466, -23.8654) (3.4396, -23.839) (3.4396, -23.8654) knots 0 0 0 0 1 1 1 1
  line L715 (3.4396, -23.8654) -> (3.4396, -25.4)
  spline S723 degree 3 poles (3.4396, -25.4) (3.4396, -25.4265) (3.466, -25.4) (3.4396, -25.4) knots 0 0 0 0 1 1 1 1
  line L716 (3.4396, -25.4) -> (2.6723, -25.4)
  spline S724 degree 3 poles (2.6723, -25.4) (2.6577, -25.4) (2.6458, -25.4119) (2.6458, -25.4265) knots 0 0 0 0 1 1 1 1
  line L717 (2.6458, -25.4265) -> (2.6458, -27.014)
  spline S725 degree 3 poles (2.6458, -27.014) (2.6458, -27.0285) (2.6577, -27.0404) (2.6723, -27.0404) knots 0 0 0 0 1 1 1 1
  line L718 (2.6723, -27.0404) -> (3.4396, -27.0404)
  spline S726 degree 3 poles (3.4396, -27.0404) (3.466, -27.0404) (3.4396, -27.014) (3.4396, -27.0404) knots 0 0 0 0 1 1 1 1
  line L719 (3.4396, -27.0404) -> (3.4396, -28.575)
  spline S727 degree 3 poles (3.4396, -28.575) (3.4396, -28.6015) (3.466, -28.575) (3.4396, -28.575) knots 0 0 0 0 1 1 1 1
  line L720 (3.4396, -28.575) -> (2.6723, -28.575)
  spline S728 degree 3 poles (2.6723, -28.575) (2.6577, -28.575) (2.6458, -28.5869) (2.6458, -28.6015) knots 0 0 0 0 1 1 1 1
  line L721 (2.6458, -28.6015) -> (2.6458, -29.9244)
  line L722 (2.6458, -29.9244) -> (2.6458, -30.7181)
  spline S729 degree 3 poles (2.6458, -30.7181) (2.6458, -30.7327) (2.6577, -30.7446) (2.6723, -30.7446) knots 0 0 0 0 1 1 1 1
  line L723 (2.6723, -30.7446) -> (3.466, -30.7446)
  line L724 (45.5612, -28.7073) -> (45.5612, -29.4746)
  spline S730 degree 3 poles (45.5612, -29.4746) (45.5612, -29.501) (45.5877, -29.4746) (45.5612, -29.4746) knots 0 0 0 0 1 1 1 1
  line L725 (45.5612, -29.4746) -> (44.8204, -29.4746)
  spline S731 degree 3 poles (44.8204, -29.4746) (44.794, -29.4746) (44.8204, -29.501) (44.8204, -29.4746) knots 0 0 0 0 1 1 1 1
  line L726 (44.8204, -29.4746) -> (44.8204, -27.94)
  spline S732 degree 3 poles (44.8204, -27.94) (44.8204, -27.9135) (44.794, -27.94) (44.8204, -27.94) knots 0 0 0 0 1 1 1 1
  line L727 (44.8204, -27.94) -> (45.5612, -27.94)
  spline S733 degree 3 poles (45.5612, -27.94) (45.5877, -27.94) (45.5612, -27.9135) (45.5612, -27.94) knots 0 0 0 0 1 1 1 1
  line L728 (45.5612, -27.94) -> (45.5612, -28.7073)
  line L729 (45.5612, -25.5323) -> (45.5612, -26.2996)
  spline S734 degree 3 poles (45.5612, -26.2996) (45.5612, -26.326) (45.5877, -26.2996) (45.5612, -26.2996) knots 0 0 0 0 1 1 1 1
  line L730 (45.5612, -26.2996) -> (44.8204, -26.2996)
  spline S735 degree 3 poles (44.8204, -26.2996) (44.794, -26.2996) (44.8204, -26.326) (44.8204, -26.2996) knots 0 0 0 0 1 1 1 1
  line L731 (44.8204, -26.2996) -> (44.8204, -24.765)
  spline S736 degree 3 poles (44.8204, -24.765) (44.8204, -24.7385) (44.794, -24.765) (44.8204, -24.765) knots 0 0 0 0 1 1 1 1
  line L732 (44.8204, -24.765) -> (45.5612, -24.765)
  spline S737 degree 3 poles (45.5612, -24.765) (45.5877, -24.765) (45.5612, -24.7385) (45.5612, -24.765) knots 0 0 0 0 1 1 1 1
  line L733 (45.5612, -24.765) -> (45.5612, -25.5323)
  line L734 (45.5612, -22.3573) -> (45.5612, -23.1246)
  spline S738 degree 3 poles (45.5612, -23.1246) (45.5612, -23.151) (45.5877, -23.1246) (45.5612, -23.1246) knots 0 0 0 0 1 1 1 1
  line L735 (45.5612, -23.1246) -> (44.8204, -23.1246)
  spline S739 degree 3 poles (44.8204, -23.1246) (44.794, -23.1246) (44.8204, -23.151) (44.8204, -23.1246) knots 0 0 0 0 1 1 1 1
  line L736 (44.8204, -23.1246) -> (44.8204, -21.59)
  spline S740 degree 3 poles (44.8204, -21.59) (44.8204, -21.5635) (44.794, -21.59) (44.8204, -21.59) knots 0 0 0 0 1 1 1 1
  line L737 (44.8204, -21.59) -> (45.5612, -21.59)
  spline S741 degree 3 poles (45.5612, -21.59) (45.5877, -21.59) (45.5612, -21.5635) (45.5612, -21.59) knots 0 0 0 0 1 1 1 1
  line L738 (45.5612, -21.59) -> (45.5612, -22.3573)
  line L739 (45.5612, -19.1823) -> (45.5612, -19.9496)
  spline S742 degree 3 poles (45.5612, -19.9496) (45.5612, -19.976) (45.5877, -19.9496) (45.5612, -19.9496) knots 0 0 0 0 1 1 1 1
  line L740 (45.5612, -19.9496) -> (44.8204, -19.9496)
  spline S743 degree 3 poles (44.8204, -19.9496) (44.794, -19.9496) (44.8204, -19.976) (44.8204, -19.9496) knots 0 0 0 0 1 1 1 1
  line L741 (44.8204, -19.9496) -> (44.8204, -18.415)
  spline S744 degree 3 poles (44.8204, -18.415) (44.8204, -18.3885) (44.794, -18.415) (44.8204, -18.415) knots 0 0 0 0 1 1 1 1
  line L742 (44.8204, -18.415) -> (45.5612, -18.415)
  spline S745 degree 3 poles (45.5612, -18.415) (45.5877, -18.415) (45.5612, -18.3885) (45.5612, -18.415) knots 0 0 0 0 1 1 1 1
  line L743 (45.5612, -18.415) -> (45.5612, -19.1823)
  line L744 (45.5612, -16.0073) -> (45.5612, -16.7746)
  spline S746 degree 3 poles (45.5612, -16.7746) (45.5612, -16.801) (45.5877, -16.7746) (45.5612, -16.7746) knots 0 0 0 0 1 1 1 1
  line L745 (45.5612, -16.7746) -> (44.8204, -16.7746)
  spline S747 degree 3 poles (44.8204, -16.7746) (44.794, -16.7746) (44.8204, -16.801) (44.8204, -16.7746) knots 0 0 0 0 1 1 1 1
  line L746 (44.8204, -16.7746) -> (44.8204, -15.24)
  spline S748 degree 3 poles (44.8204, -15.24) (44.8204, -15.2135) (44.794, -15.24) (44.8204, -15.24) knots 0 0 0 0 1 1 1 1
  line L747 (44.8204, -15.24) -> (45.5612, -15.24)
  spline S749 degree 3 poles (45.5612, -15.24) (45.5877, -15.24) (45.5612, -15.2135) (45.5612, -15.24) knots 0 0 0 0 1 1 1 1
  line L748 (45.5612, -15.24) -> (45.5612, -16.0073)
  line L749 (45.5612, -12.8323) -> (45.5612, -13.5996)
  spline S750 degree 3 poles (45.5612, -13.5996) (45.5612, -13.626) (45.5877, -13.5996) (45.5612, -13.5996) knots 0 0 0 0 1 1 1 1
  line L750 (45.5612, -13.5996) -> (44.8204, -13.5996)
  spline S751 degree 3 poles (44.8204, -13.5996) (44.794, -13.5996) (44.8204, -13.626) (44.8204, -13.5996) knots 0 0 0 0 1 1 1 1
  line L751 (44.8204, -13.5996) -> (44.8204, -12.065)
  spline S752 degree 3 poles (44.8204, -12.065) (44.8204, -12.0385) (44.794, -12.065) (44.8204, -12.065) knots 0 0 0 0 1 1 1 1
  line L752 (44.8204, -12.065) -> (45.5612, -12.065)
  spline S753 degree 3 poles (45.5612, -12.065) (45.5877, -12.065) (45.5612, -12.0385) (45.5612, -12.065) knots 0 0 0 0 1 1 1 1
  line L753 (45.5612, -12.065) -> (45.5612, -12.8323)
  line L754 (45.5612, -9.6573) -> (45.5612, -10.4246)
  spline S754 degree 3 poles (45.5612, -10.4246) (45.5612, -10.451) (45.5877, -10.4246) (45.5612, -10.4246) knots 0 0 0 0 1 1 1 1
  line L755 (45.5612, -10.4246) -> (44.8204, -10.4246)
  spline S755 degree 3 poles (44.8204, -10.4246) (44.794, -10.4246) (44.8204, -10.451) (44.8204, -10.4246) knots 0 0 0 0 1 1 1 1
  line L756 (44.8204, -10.4246) -> (44.8204, -8.89)
  spline S756 degree 3 poles (44.8204, -8.89) (44.8204, -8.8635) (44.794, -8.89) (44.8204, -8.89) knots 0 0 0 0 1 1 1 1
  line L757 (44.8204, -8.89) -> (45.5612, -8.89)
  spline S757 degree 3 poles (45.5612, -8.89) (45.5877, -8.89) (45.5612, -8.8635) (45.5612, -8.89) knots 0 0 0 0 1 1 1 1
  line L758 (45.5612, -8.89) -> (45.5612, -9.6573)
  line L759 (45.5612, -6.4823) -> (45.5612, -7.2496)
  spline S758 degree 3 poles (45.5612, -7.2496) (45.5612, -7.276) (45.5877, -7.2496) (45.5612, -7.2496) knots 0 0 0 0 1 1 1 1
  line L760 (45.5612, -7.2496) -> (44.8204, -7.2496)
  spline S759 degree 3 poles (44.8204, -7.2496) (44.794, -7.2496) (44.8204, -7.276) (44.8204, -7.2496) knots 0 0 0 0 1 1 1 1
  line L761 (44.8204, -7.2496) -> (44.8204, -5.715)
  spline S760 degree 3 poles (44.8204, -5.715) (44.8204, -5.6885) (44.794, -5.715) (44.8204, -5.715) knots 0 0 0 0 1 1 1 1
  line L762 (44.8204, -5.715) -> (45.5612, -5.715)
  spline S761 degree 3 poles (45.5612, -5.715) (45.5877, -5.715) (45.5612, -5.6885) (45.5612, -5.715) knots 0 0 0 0 1 1 1 1
  line L763 (45.5612, -5.715) -> (45.5612, -6.4823)
  line L764 (44.3971, -30.7446) -> (45.9846, -30.7446)
  line L765 (45.9846, -30.7446) -> (92.5068, -30.7446)
  spline S762 degree 3 poles (92.5068, -30.7446) (92.5214, -30.7446) (92.5333, -30.7327) (92.5333, -30.7181) knots 0 0 0 0 1 1 1 1
  line L766 (92.5333, -30.7181) -> (92.5333, -4.4185)
  spline S763 degree 3 poles (92.5333, -4.4185) (92.5333, -4.404) (92.5214, -4.3921) (92.5068, -4.3921) knots 0 0 0 0 1 1 1 1
  line L767 (92.5068, -4.3921) -> (44.3971, -4.3921)
  spline S764 degree 3 poles (44.3971, -4.3921) (44.3825, -4.3921) (44.3706, -4.404) (44.3706, -4.4185) knots 0 0 0 0 1 1 1 1
  line L768 (44.3706, -4.4185) -> (44.3706, -30.7181)
  spline S765 degree 3 poles (44.3706, -30.7181) (44.3706, -30.7327) (44.3825, -30.7446) (44.3971, -30.7446) knots 0 0 0 0 1 1 1 1
  line L769 (46.6238, -30.7446) -> (46.6238, -26.6171)
  line L770 (46.6238, -25.0296) -> (46.6238, -18.3621)
  line L771 (46.6238, -16.7746) -> (46.6238, -10.1071)
  line L772 (46.6238, -8.5196) -> (46.6238, -4.3921)
  line L773 (47.2191, -5.9796) -> (47.2191, -12.6471)
  line L774 (47.2191, -14.2346) -> (47.2191, -20.9021)
  line L775 (47.2191, -22.4896) -> (47.2191, -29.1571)
  line L776 (47.8144, -30.7446) -> (47.8144, -26.6171)
  line L777 (47.8144, -25.0296) -> (47.8144, -18.3621)
  line L778 (47.8144, -16.7746) -> (47.8144, -10.1071)
  line L779 (47.8144, -8.5196) -> (47.8144, -4.3921)
  line L780 (48.4098, -5.9796) -> (48.4098, -12.6471)
  line L781 (48.4098, -14.2346) -> (48.4098, -20.9021)
  line L782 (48.4098, -22.4896) -> (48.4098, -29.1571)
  line L783 (49.0051, -30.7446) -> (49.0051, -26.6171)
  line L784 (49.0051, -25.0296) -> (49.0051, -18.3621)
  line L785 (49.0051, -16.7746) -> (49.0051, -10.1071)
  line L786 (49.0051, -8.5196) -> (49.0051, -4.3921)
  line L787 (49.6004, -5.9796) -> (49.6004, -12.6471)
  line L788 (49.6004, -14.2346) -> (49.6004, -20.9021)
  line L789 (49.6004, -22.4896) -> (49.6004, -29.1571)
  line L790 (50.1957, -30.7446) -> (50.1957, -26.6171)
  line L791 (50.1957, -25.0296) -> (50.1957, -18.3621)
  line L792 (50.1957, -16.7746) -> (50.1957, -10.1071)
  line L793 (50.1957, -8.5196) -> (50.1957, -4.3921)
  line L794 (50.791, -5.9796) -> (50.791, -12.6471)
  line L795 (50.791, -14.2346) -> (50.791, -20.9021)
  line L796 (50.791, -22.4896) -> (50.791, -29.1571)
  line L797 (51.3863, -30.7446) -> (51.3863, -26.6171)
  line L798 (51.3863, -25.0296) -> (51.3863, -18.3621)
  line L799 (51.3863, -16.7746) -> (51.3863, -10.1071)
  line L800 (51.3863, -8.5196) -> (51.3863, -4.3921)
  line L801 (51.9816, -5.9796) -> (51.9816, -12.6471)
  line L802 (51.9816, -14.2346) -> (51.9816, -20.9021)
  line L803 (51.9816, -22.4896) -> (51.9816, -29.1571)
  line L804 (52.5769, -30.7446) -> (52.5769, -26.6171)
  line L805 (52.5769, -25.0296) -> (52.5769, -18.3621)
  line L806 (52.5769, -16.7746) -> (52.5769, -10.1071)
  line L807 (52.5769, -8.5196) -> (52.5769, -4.3921)
  line L808 (53.1723, -5.9796) -> (53.1723, -12.6471)
  line L809 (53.1723, -14.2346) -> (53.1723, -20.9021)
  line L810 (53.1723, -22.4896) -> (53.1723, -29.1571)
  line L811 (53.7676, -30.7446) -> (53.7676, -26.6171)
  line L812 (53.7676, -25.0296) -> (53.7676, -18.3621)
  line L813 (53.7676, -16.7746) -> (53.7676, -10.1071)
  line L814 (53.7676, -8.5196) -> (53.7676, -4.3921)
  line L815 (54.3629, -5.9796) -> (54.3629, -12.6471)
  line L816 (54.3629, -14.2346) -> (54.3629, -20.9021)
  line L817 (54.3629, -22.4896) -> (54.3629, -29.1571)
  line L818 (54.9582, -30.7446) -> (54.9582, -26.6171)
  line L819 (54.9582, -25.0296) -> (54.9582, -18.3621)
  line L820 (54.9582, -16.7746) -> (54.9582, -10.1071)
  line L821 (54.9582, -8.5196) -> (54.9582, -4.3921)
  line L822 (55.5535, -5.9796) -> (55.5535, -12.6471)
  line L823 (55.5535, -14.2346) -> (55.5535, -20.9021)
  line L824 (55.5535, -22.4896) -> (55.5535, -29.1571)
  line L825 (56.1488, -30.7446) -> (56.1488, -26.6171)
  line L826 (56.1488, -25.0296) -> (56.1488, -18.3621)
  line L827 (56.1488, -16.7746) -> (56.1488, -10.1071)
  line L828 (56.1488, -8.5196) -> (56.1488, -4.3921)
  line L829 (56.7441, -5.9796) -> (56.7441, -12.6471)
  line L830 (56.7441, -14.2346) -> (56.7441, -20.9021)
  line L831 (56.7441, -22.4896) -> (56.7441, -29.1571)
  line L832 (57.3394, -30.7446) -> (57.3394, -26.6171)
  line L833 (57.3394, -25.0296) -> (57.3394, -18.3621)
  line L834 (57.3394, -16.7746) -> (57.3394, -10.1071)
  line L835 (57.3394, -8.5196) -> (57.3394, -4.3921)
  line L836 (57.9348, -5.9796) -> (57.9348, -12.6471)
  line L837 (57.9348, -14.2346) -> (57.9348, -20.9021)
  line L838 (57.9348, -22.4896) -> (57.9348, -29.1571)
  line L839 (58.5301, -30.7446) -> (58.5301, -26.6171)
  line L840 (58.5301, -25.0296) -> (58.5301, -18.3621)
  line L841 (58.5301, -16.7746) -> (58.5301, -10.1071)
  line L842 (58.5301, -8.5196) -> (58.5301, -4.3921)
  line L843 (59.1254, -5.9796) -> (59.1254, -12.6471)
  line L844 (59.1254, -14.2346) -> (59.1254, -20.9021)
  line L845 (59.1254, -22.4896) -> (59.1254, -29.1571)
  line L846 (59.7207, -30.7446) -> (59.7207, -26.6171)
  line L847 (59.7207, -25.0296) -> (59.7207, -18.3621)
  line L848 (59.7207, -16.7746) -> (59.7207, -10.1071)
  line L849 (59.7207, -8.5196) -> (59.7207, -4.3921)
  line L850 (60.316, -5.9796) -> (60.316, -12.6471)
  line L851 (60.316, -14.2346) -> (60.316, -20.9021)
  line L852 (60.316, -22.4896) -> (60.316, -29.1571)
  line L853 (60.9113, -30.7446) -> (60.9113, -26.6171)
  line L854 (60.9113, -25.0296) -> (60.9113, -18.3621)
  line L855 (60.9113, -16.7746) -> (60.9113, -10.1071)
  line L856 (60.9113, -8.5196) -> (60.9113, -4.3921)
  line L857 (61.5066, -5.9796) -> (61.5066, -12.6471)
  line L858 (61.5066, -14.2346) -> (61.5066, -20.9021)
  line L859 (61.5066, -22.4896) -> (61.5066, -29.1571)
  line L860 (62.1019, -30.7446) -> (62.1019, -26.6171)
  line L861 (62.1019, -25.0296) -> (62.1019, -18.3621)
  line L862 (62.1019, -16.7746) -> (62.1019, -10.1071)
  line L863 (62.1019, -8.5196) -> (62.1019, -4.3921)
  line L864 (62.6973, -5.9796) -> (62.6973, -12.6471)
  line L865 (62.6973, -14.2346) -> (62.6973, -20.9021)
  line L866 (62.6973, -22.4896) -> (62.6973, -29.1571)
  line L867 (63.2926, -30.7446) -> (63.2926, -26.6171)
  line L868 (63.2926, -25.0296) -> (63.2926, -18.3621)
  line L869 (63.2926, -16.7746) -> (63.2926, -10.1071)
  line L870 (63.2926, -8.5196) -> (63.2926, -4.3921)
  line L871 (63.8879, -5.9796) -> (63.8879, -12.6471)
  line L872 (63.8879, -14.2346) -> (63.8879, -20.9021)
  line L873 (63.8879, -22.4896) -> (63.8879, -29.1571)
  line L874 (64.4832, -30.7446) -> (64.4832, -26.6171)
  line L875 (64.4832, -25.0296) -> (64.4832, -18.3621)
  line L876 (64.4832, -16.7746) -> (64.4832, -10.1071)
  line L877 (64.4832, -8.5196) -> (64.4832, -4.3921)
  line L878 (65.0785, -5.9796) -> (65.0785, -12.6471)
  line L879 (65.0785, -14.2346) -> (65.0785, -20.9021)
  line L880 (65.0785, -22.4896) -> (65.0785, -29.1571)
  line L881 (65.6738, -30.7446) -> (65.6738, -26.6171)
  line L882 (65.6738, -25.0296) -> (65.6738, -18.3621)
  line L883 (65.6738, -16.7746) -> (65.6738, -10.1071)
  line L884 (65.6738, -8.5196) -> (65.6738, -4.3921)
  line L885 (66.2691, -5.9796) -> (66.2691, -12.6471)
  line L886 (66.2691, -14.2346) -> (66.2691, -20.9021)
  line L887 (66.2691, -22.4896) -> (66.2691, -29.1571)
  line L888 (66.8644, -30.7446) -> (66.8644, -26.6171)
  line L889 (66.8644, -25.0296) -> (66.8644, -18.3621)
  line L890 (66.8644, -16.7746) -> (66.8644, -10.1071)
  line L891 (66.8644, -8.5196) -> (66.8644, -4.3921)
  line L892 (67.4598, -5.9796) -> (67.4598, -12.6471)
  line L893 (67.4598, -14.2346) -> (67.4598, -20.9021)
  line L894 (67.4598, -22.4896) -> (67.4598, -29.1571)
  line L895 (68.0551, -30.7446) -> (68.0551, -26.6171)
  line L896 (68.0551, -25.0296) -> (68.0551, -18.3621)
  line L897 (68.0551, -16.7746) -> (68.0551, -10.1071)
  line L898 (68.0551, -8.5196) -> (68.0551, -4.3921)
  line L899 (68.6504, -5.9796) -> (68.6504, -12.6471)
  line L900 (68.6504, -14.2346) -> (68.6504, -20.9021)
  line L901 (68.6504, -22.4896) -> (68.6504, -29.1571)
  line L902 (69.2457, -30.7446) -> (69.2457, -26.6171)
  line L903 (69.2457, -25.0296) -> (69.2457, -18.3621)
  line L904 (69.2457, -16.7746) -> (69.2457, -10.1071)
  line L905 (69.2457, -8.5196) -> (69.2457, -4.3921)
  line L906 (69.841, -5.9796) -> (69.841, -12.6471)
  line L907 (69.841, -14.2346) -> (69.841, -20.9021)
  line L908 (69.841, -22.4896) -> (69.841, -29.1571)
  line L909 (70.4363, -30.7446) -> (70.4363, -26.6171)
  line L910 (70.4363, -25.0296) -> (70.4363, -18.3621)
  line L911 (70.4363, -16.7746) -> (70.4363, -10.1071)
  line L912 (70.4363, -8.5196) -> (70.4363, -4.3921)
  line L913 (71.0316, -5.9796) -> (71.0316, -12.6471)
  line L914 (71.0316, -14.2346) -> (71.0316, -20.9021)